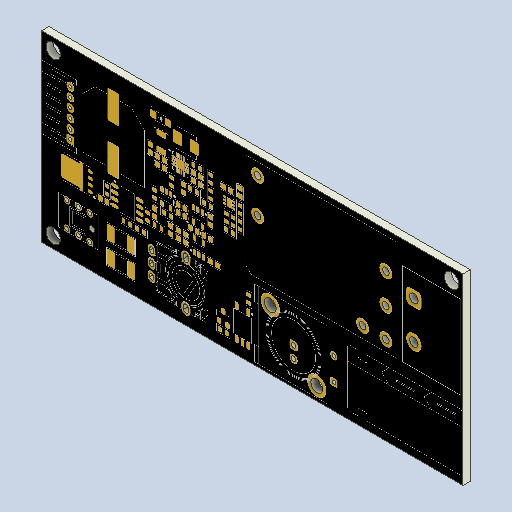
# Autodesk Inventor part: Monitor_Blanking_V3_BOARD
Saved by Autodesk Inventor 2025.3 (Build 293356000, 356)
## iProperties
Created: 2025-06-10
Part Number: Monitor_Blanking_V3_BOARD
Material: Generic
Document SubType Name: Modeling
Designer: Yuhsuan Chen
Density: 1 g/cm^3
Appearance: BoardColor
Author: Yuhsuan Chen
Autodesk Inventor part; units mm, degrees
ref_plane "YZ Plane" through (0, 0, 0) normal (1, 0, 0) x (0, 1, 0)
ref_plane "XZ Plane" through (0, 0, 0) normal (0, 1, 0) x (-1, 0, 0)
ref_plane "XY Plane" through (0, 0, 0) normal (0, 0, 1) x (1, 0, 0)
ref_plane "BoardFrontPlane" through (0, 0, 0) normal (0, 0, 1) x (1, 0, 0)
sketch "Sketch1" plane through (0, 0, 0) normal (0, 0, 1) x (1, 0, 0)
  line L0 (149.925, 120.925) -> (241.925, 120.925)
  line L1 (241.925, 120.925) -> (241.925, 160.925)
  line L2 (241.925, 160.925) -> (149.925, 160.925)
  line L3 (149.925, 160.925) -> (149.925, 120.925)
  constraints: 8 end point
extrude "BoardOutline" add sketch "Sketch1" along normal blind 1.5954
sketch "img_Top" plane through (0, 0, 1.5954) normal (0, 0, 1) x (1, 0, 0)
  line L0 (149.925, 160.925) -> (241.925, 160.925) construction
  line L1 (241.925, 160.925) -> (241.925, 120.9195) construction
  line L2 (241.925, 120.9195) -> (149.925, 120.9195) construction
  line L3 (149.925, 120.9195) -> (149.925, 160.925) construction
  constraints: 2 other
decal "Decal_Top"
sketch "img_Bottom" plane through (0, 0, -1.5954) normal (0, 0, -1) x (1, 0, 0)
  line L0 (149.925, -120.925) -> (241.925, -120.925) construction
  line L1 (241.925, -120.925) -> (241.925, -160.9305) construction
  line L2 (241.925, -160.9305) -> (149.925, -160.9305) construction
  line L3 (149.925, -160.9305) -> (149.925, -120.925) construction
  constraints: 2 other
decal "Decal_Bottom"
sketch "Sketch4" plane through (0, 0, 1.5954) normal (0, 0, 1) x (1, 0, 0)
  point P0 (219.993, 140.177)
hole "U1-1" at (219.993, 140.177, 1.5954) direction (0, 0, -1) diameter 1.5 end through all
sketch "Sketch5" plane through (0, 0, 1.5954) normal (0, 0, 1) x (1, 0, 0)
  point P0 (225.073, 153.027)
hole "U1-4" at (225.073, 153.027, 1.5954) direction (0, 0, -1) diameter 1.5 end through all
sketch "Sketch6" plane through (0, 0, 1.5954) normal (0, 0, 1) x (1, 0, 0)
  point P0 (225.073, 146.527)
hole "U1-3" at (225.073, 146.527, 1.5954) direction (0, 0, -1) diameter 1.5 end through all
sketch "Sketch7" plane through (0, 0, 1.5954) normal (0, 0, 1) x (1, 0, 0)
  point P0 (197.073, 157.127)
hole "U1-5" at (197.073, 157.127, 1.5954) direction (0, 0, -1) diameter 1.5 end through all
sketch "Sketch8" plane through (0, 0, 1.5954) normal (0, 0, 1) x (1, 0, 0)
  point P0 (197.073, 149.507)
hole "U1-6" at (197.073, 149.507, 1.5954) direction (0, 0, -1) diameter 1.5 end through all
sketch "Sketch9" plane through (0, 0, 1.5954) normal (0, 0, 1) x (1, 0, 0)
  point P0 (225.073, 140.127)
hole "U1-2" at (225.073, 140.127, 1.5954) direction (0, 0, -1) diameter 1.5 end through all
sketch "Sketch10" plane through (0, 0, 1.5954) normal (0, 0, 1) x (1, 0, 0)
  point P0 (155.425, 126.225)
hole "SW1-1" at (155.425, 126.225, 1.5954) direction (0, 0, -1) diameter 0.9 end through all
sketch "Sketch11" plane through (0, 0, 1.5954) normal (0, 0, 1) x (1, 0, 0)
  point P0 (157.925, 126.225)
hole "SW1-2" at (157.925, 126.225, 1.5954) direction (0, 0, -1) diameter 0.9 end through all
sketch "Sketch12" plane through (0, 0, 1.5954) normal (0, 0, 1) x (1, 0, 0)
  point P0 (160.425, 126.225)
hole "SW1-3" at (160.425, 126.225, 1.5954) direction (0, 0, -1) diameter 0.9 end through all
sketch "Sketch13" plane through (0, 0, 1.5954) normal (0, 0, 1) x (1, 0, 0)
  point P0 (157.925, 131.625)
hole "SW1-5" at (157.925, 131.625, 1.5954) direction (0, 0, -1) diameter 0.9 end through all
sketch "Sketch14" plane through (0, 0, 1.5954) normal (0, 0, 1) x (1, 0, 0)
  point P0 (160.425, 131.625)
hole "SW1-6" at (160.425, 131.625, 1.5954) direction (0, 0, -1) diameter 0.9 end through all
sketch "Sketch15" plane through (0, 0, 1.5954) normal (0, 0, 1) x (1, 0, 0)
  point P0 (155.425, 131.625)
hole "SW1-4" at (155.425, 131.625, 1.5954) direction (0, 0, -1) diameter 0.9 end through all
sketch "Sketch16" plane through (0, 0, 1.5954) normal (0, 0, 1) x (1, 0, 0)
  point P0 (160.925, 128.925)
hole "SW1-0" at (160.925, 128.925, 1.5954) direction (0, 0, -1) diameter 1.2 end through all
sketch "Sketch22" plane through (0, 0, 1.5954) normal (0, 0, 1) x (1, 0, 0)
  point P0 (156.175, 143.45)
hole "CN2-1" at (156.175, 143.45, 1.5954) direction (0, 0, -1) diameter 0.72 end through all
sketch "Sketch23" plane through (0, 0, 1.5954) normal (0, 0, 1) x (1, 0, 0)
  point P0 (156.175, 149.45)
hole "CN2-4" at (156.175, 149.45, 1.5954) direction (0, 0, -1) diameter 0.72 end through all
sketch "Sketch24" plane through (0, 0, 1.5954) normal (0, 0, 1) x (1, 0, 0)
  point P0 (156.175, 145.45)
hole "CN2-2" at (156.175, 145.45, 1.5954) direction (0, 0, -1) diameter 0.72 end through all
sketch "Sketch25" plane through (0, 0, 1.5954) normal (0, 0, 1) x (1, 0, 0)
  point P0 (156.175, 151.45)
hole "CN2-5" at (156.175, 151.45, 1.5954) direction (0, 0, -1) diameter 0.72 end through all
sketch "Sketch26" plane through (0, 0, 1.5954) normal (0, 0, 1) x (1, 0, 0)
  point P0 (156.175, 147.45)
hole "CN2-3" at (156.175, 147.45, 1.5954) direction (0, 0, -1) diameter 0.72 end through all
sketch "Sketch27" plane through (0, 0, 1.5954) normal (0, 0, 1) x (1, 0, 0)
  point P0 (156.175, 153.45)
hole "CN2-6" at (156.175, 153.45, 1.5954) direction (0, 0, -1) diameter 0.72 end through all
sketch "Sketch28" plane through (0, 0, 1.5954) normal (0, 0, 1) x (1, 0, 0)
  point P0 (231.2, 150.95)
hole "CN1-1" at (231.2, 150.95, 1.5954) direction (0, 0, -1) diameter 1.9 end through all
sketch "Sketch29" plane through (0, 0, 1.5954) normal (0, 0, 1) x (1, 0, 0)
  point P0 (231.2, 142.69)
hole "CN1-2" at (231.2, 142.69, 1.5954) direction (0, 0, -1) diameter 1.9 end through all
sketch "Sketch30" plane through (0, 0, 1.5954) normal (0, 0, 1) x (1, 0, 0)
  point P0 (213.725, 126.35)
hole "C2-1" at (213.725, 126.35, 1.5954) direction (0, 0, -1) diameter 0.8 end through all
sketch "Sketch31" plane through (0, 0, 1.5954) normal (0, 0, 1) x (1, 0, 0)
  point P0 (213.725, 131.35)
hole "C2-2" at (213.725, 131.35, 1.5954) direction (0, 0, -1) diameter 0.8 end through all
sketch "Sketch32" plane through (0, 0, 1.5954) normal (0, 0, 1) x (1, 0, 0)
  point P0 (204.925, 128.925)
hole "CN3-1" at (204.925, 128.925, 1.5954) direction (0, 0, -1) diameter 1 end through all
sketch "Sketch33" plane through (0, 0, 1.5954) normal (0, 0, 1) x (1, 0, 0)
  point P0 (199.845, 134.005)
hole "CN3-2_KIXDPQYP" at (199.845, 134.005, 1.5954) direction (0, 0, -1) diameter 2.64 end through all
sketch "Sketch34" plane through (0, 0, 1.5954) normal (0, 0, 1) x (1, 0, 0)
  point P0 (210.005, 123.845)
hole "CN3-2_CBVBVUTG" at (210.005, 123.845, 1.5954) direction (0, 0, -1) diameter 2.64 end through all
sketch "Sketch35" plane through (0, 0, 1.5954) normal (0, 0, 1) x (1, 0, 0)
  point P0 (204.925, 126.385)
hole "CN3-2_RGICKRHG" at (204.925, 126.385, 1.5954) direction (0, 0, -1) diameter 1 end through all
sketch "Sketch36" plane through (0, 0, 1.5954) normal (0, 0, 1) x (1, 0, 0)
  point P0 (239.425, 158.425)
hole "Free-0_VQVYAAFI" at (239.425, 158.425, 1.5954) direction (0, 0, -1) diameter 3.2 end through all
sketch "Sketch37" plane through (0, 0, 1.5954) normal (0, 0, 1) x (1, 0, 0)
  point P0 (152.425, 123.425)
hole "Free-0_TSXFHYQJ" at (152.425, 123.425, 1.5954) direction (0, 0, -1) diameter 3.2 end through all
sketch "Sketch38" plane through (0, 0, 1.5954) normal (0, 0, 1) x (1, 0, 0)
  point P0 (152.425, 158.425)
hole "Free-0_JLGAYVLC" at (152.425, 158.425, 1.5954) direction (0, 0, -1) diameter 3.2 end through all
sketch "Sketch54" plane through (0, 0, 1.5954) normal (0, 0, 1) x (1, 0, 0)
  line L0 (181.425, 133.3251) -> (181.425, 134.1251) construction
  line L1 (181.925, 133.3251) -> (181.925, 134.1251)
  line L2 (180.925, 134.1251) -> (180.925, 133.3251)
  arc A0 (180.925, 133.3251) -> (181.925, 133.3251) centre (181.425, 133.3251) ccw
  arc A1 (181.925, 134.1251) -> (180.925, 134.1251) centre (181.425, 134.1251) ccw
  point P0 (181.425, 133.7251)
  constraints: 8 end point, 4 point on circle, 4 tangent, 2 centre point, 1 midpoint, 1 parallel
extrude "R3-0_UKQXETQG" cut sketch "Sketch54" against normal through all
sketch "Sketch55" plane through (0, 0, 1.5954) normal (0, 0, 1) x (1, 0, 0)
  line L0 (181.425, 123.7251) -> (181.425, 124.5251) construction
  line L1 (181.925, 123.7251) -> (181.925, 124.5251)
  line L2 (180.925, 124.5251) -> (180.925, 123.7251)
  arc A0 (180.925, 123.7251) -> (181.925, 123.7251) centre (181.425, 123.7251) ccw
  arc A1 (181.925, 124.5251) -> (180.925, 124.5251) centre (181.425, 124.5251) ccw
  point P0 (181.425, 124.1251)
  constraints: 8 end point, 4 point on circle, 4 tangent, 2 centre point, 1 midpoint, 1 parallel
extrude "R3-0_WDTRLAVX" cut sketch "Sketch55" against normal through all
sketch "Sketch56" plane through (0, 0, 1.5954) normal (0, 0, 1) x (1, 0, 0)
  line L0 (173.925, 131.19) -> (173.925, 131.6601) construction
  line L1 (174.325, 131.19) -> (174.325, 131.6601)
  line L2 (173.525, 131.6601) -> (173.525, 131.19)
  arc A0 (173.525, 131.19) -> (174.325, 131.19) centre (173.925, 131.19) ccw
  arc A1 (174.325, 131.6601) -> (173.525, 131.6601) centre (173.925, 131.6601) ccw
  point P0 (173.925, 131.425)
  constraints: 8 end point, 4 point on circle, 4 tangent, 2 centre point, 1 midpoint, 1 parallel
extrude "R3-1" cut sketch "Sketch56" against normal through all
sketch "Sketch57" plane through (0, 0, 1.5954) normal (0, 0, 1) x (1, 0, 0)
  line L0 (173.925, 126.1901) -> (173.925, 126.6601) construction
  line L1 (174.325, 126.1901) -> (174.325, 126.6601)
  line L2 (173.525, 126.6601) -> (173.525, 126.1901)
  arc A0 (173.525, 126.1901) -> (174.325, 126.1901) centre (173.925, 126.1901) ccw
  arc A1 (174.325, 126.6601) -> (173.525, 126.6601) centre (173.925, 126.6601) ccw
  point P0 (173.925, 126.4251)
  constraints: 8 end point, 4 point on circle, 4 tangent, 2 centre point, 1 midpoint, 1 parallel
extrude "R3-3" cut sketch "Sketch57" against normal through all
sketch "Sketch58" plane through (0, 0, 1.5954) normal (0, 0, 1) x (1, 0, 0)
  line L0 (173.925, 128.69) -> (173.925, 129.1601) construction
  line L1 (174.325, 128.69) -> (174.325, 129.1601)
  line L2 (173.525, 129.1601) -> (173.525, 128.69)
  arc A0 (173.525, 128.69) -> (174.325, 128.69) centre (173.925, 128.69) ccw
  arc A1 (174.325, 129.1601) -> (173.525, 129.1601) centre (173.925, 129.1601) ccw
  point P0 (173.925, 128.925)
  constraints: 8 end point, 4 point on circle, 4 tangent, 2 centre point, 1 midpoint, 1 parallel
extrude "R3-2" cut sketch "Sketch58" against normal through all
body "Solid1"
